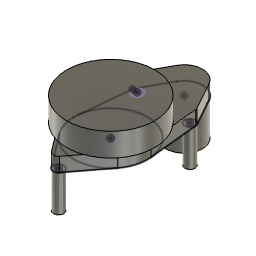
Lidar v1 (Autodesk Fusion 360 design; units mm, degrees)
Autodesk Fusion 360 part; units mm, degrees
sketch "Sketch1" plane through (0, 0, 0) normal (0, 0, 1) x (1, 0, 0)
  circle A0 centre (0, 0) radius 3.5
  circle A1 centre (-18, 71.5) radius 3.5
  circle A2 centre (18, 71.5) radius 3.5
  circle A3 centre (0, 85.5) radius 12.5
  line L0 (-18, 71.5) -> (18, 71.5) construction
  line L1 (0, 85.5) -> (0, 0) construction
  circle A4 centre (0, 35.5) radius 30.25
  dimension "d1" = 36
  dimension "d2" = 18
  dimension "d3" = 7
  dimension "d4" = 7
  dimension "d5" = 7
  dimension "d6" = 25
  dimension "d7" = 60.5
  dimension "d8" = 35.5
  dimension "d9" = 36
  dimension "d10" = 50
  constraint coincident A0.centre L1.end
  constraint coincident A1.centre L0.start
  constraint coincident A2.centre L0.end
  constraint horizontal L0
  constraint coincident A3.centre L1.start
  constraint vertical L1
  constraint coincident L1 A4.centre
  measures "d1" distance of A1.centre A2.centre
  measures "d2" distance of A2.centre L1
  measures "d3" diameter of A1
  measures "d4" diameter of A2
  measures "d5" diameter of A0
  measures "d6" diameter of A3
  measures "d7" diameter of A4
  measures "d8" distance of A0.centre A4.centre
  measures "d9" distance of L0 A4.centre
  measures "d10" distance of A3.centre A4.centre
extrude "Extrude1" add sketch "Sketch1" along normal blind 25 contours A0 | A1 | A2 | A3 makes body 1 at (14.9262, 69.8261, 16.6667) makes body 2 at (3.4826, -0.3485, 8.3333) makes body 3 at (-14.7111, 70.3029, 16.6667) makes body 4 at (12.4379, 84.2554, 8.3333)
sketch "Sketch2" plane through (0, 0, 25) normal (0, 0, 1) x (-1, 0, 0)
  circle A0 centre (0, -85.5) radius 12.5
  circle A1 centre (-18, -71.5) radius 3.5
  circle A2 centre (0, -35.5) radius 25
  line L0 (10.9455, -91.5371) -> (21.0647, -73.1904)
  line L1 (-10.9455, -91.5371) -> (-21.0647, -73.1904)
  circle A3 centre (0, 0) radius 3.5
  line L2 (21.4826, -71.849) -> (24.8754, -37.9929)
  line L3 (-21.4826, -71.849) -> (-24.8754, -37.9929)
  line L4 (2.7851, 2.1197) -> (19.8936, -20.3592)
  line L5 (-2.7851, 2.1197) -> (-19.8936, -20.3592)
  arc A4 (21.0647, -73.1904) -> (21.4826, -71.849) centre (18, -71.5) ccw
  arc A5 (-10.9455, -91.5371) -> (10.9455, -91.5371) centre (0, -85.5) ccw
  circle A6 centre (18, -71.5) radius 3.5
  point P0 (18, -71.5)
  point P1 (-18, -71.5)
  point P2 (0, -35.5)
  dimension "d13" = 7
  dimension "d14" = 7
  dimension "d15" = 25
  dimension "d16" = 7
  dimension "d17" = 50
  constraint concentric A0 A5
  constraint tangent L0 A4
  constraint tangent A1 L1
  constraint tangent L0 A5
  constraint tangent L1 A5
  constraint coincident P0 A4.centre
  constraint coincident P1 A1.centre
  constraint coincident A3.centre origin
  constraint coincident P2 A2.centre
  constraint coincident A2 L2.end
  constraint coincident A2 L3.end
  constraint coincident A3 L4.start
  constraint coincident A2 L4.end
  constraint coincident A3 L5.start
  constraint coincident A2 L5.end
  constraint tangent A2 L3
  constraint tangent A1 L3
  constraint tangent L2 A4
  constraint tangent A2 L2
  constraint tangent A2 L4
  constraint tangent A2 L5
  constraint tangent A3 L5
  constraint tangent A3 L4
  constraint coincident L2 A4.end
  constraint coincident A1 L1.end
  constraint coincident A1 L3.start
  constraint coincident L2.start A6
  measures "d13" diameter of A4
  measures "d14" diameter of A1
  measures "d15" diameter of A5
  measures "d16" diameter of A3
  measures "d17" diameter of A2
extrude "Extrude2" add sketch "Sketch2" 1 faces at (-18.2596, 72.6374, 25) along normal blind 9.5 contours A0 A5 | A1 | A2 | A2 A3 L4 L5 | A3 on bodies 3 bodies 3 1 2 4
extrude "Extrude3" add sketch "Sketch2" along normal blind 9.5 contours A0 A1 A2 L0 L1 L2 L3 A6 bodies 1 2 3 4
sketch "Sketch4" plane through (0, 0, 34.5) normal (0, 0, 1) x (-1, 0, 0)
  arc A0 (21.0647, -73.1904) -> (21.4826, -71.849) centre (18, -71.5) ccw
  line L0 (21.4826, -71.849) -> (24.8754, -37.9929)
  arc A1 (24.8754, -37.9929) -> (19.8936, -20.3592) centre (0, -35.5) ccw
  line L1 (19.8936, -20.3592) -> (2.7851, 2.1197)
  arc A2 (2.7851, 2.1197) -> (-2.7851, 2.1197) centre (0, 0) ccw
  line L2 (-2.7851, 2.1197) -> (-19.8936, -20.3592)
  arc A3 (-19.8936, -20.3592) -> (-24.8754, -37.9929) centre (0, -35.5) ccw
  line L3 (-24.8754, -37.9929) -> (-21.4826, -71.849)
  arc A4 (-21.4826, -71.849) -> (-21.0647, -73.1904) centre (-18, -71.5) ccw
  line L4 (-21.0647, -73.1904) -> (-10.9455, -91.5371)
  arc A5 (-10.9455, -91.5371) -> (10.9455, -91.5371) centre (0, -85.5) ccw
  line L5 (10.9455, -91.5371) -> (21.0647, -73.1904)
  circle A6 centre (0, -35.5) radius 30
  dimension "d22" = 60
  constraint concentric A1 A6
  measures "d22" diameter of A6
extrude "Extrude4" add sketch "Sketch4" along normal blind 15.8 contours L0 A1 L1 L2 A3 L3 A6 | L0 A1 L1 A6 | L2 A3 L3 A6 bodies 1
